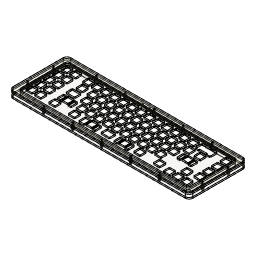
FrogdorCase (Autodesk Fusion 360 design; units mm, degrees)
Autodesk Fusion 360 part; units mm, degrees
(part 1 of 3)
sketch "Frogdor Top Plate" plane through (0, 0, 0) normal (0, 0, 1) x (1, 0, 0)
  line L0 (107.3, -7.3375) -> (107.3, -19.3375)
  line L1 (22.575, -39.3875) -> (34.575, -39.3875)
  arc A0 (184.5, -6.3375) -> (183.5, -7.3375) centre (184.5, -7.3375) ccw
  line L2 (279.75, -6.3375) -> (291.75, -6.3375)
  arc A1 (102.25, -7.3375) -> (101.25, -6.3375) centre (101.25, -7.3375) ccw
  arc A2 (221.6, -19.3375) -> (222.6, -20.3375) centre (222.6, -19.3375) ccw
  arc A3 (183.5, -19.3375) -> (184.5, -20.3375) centre (184.5, -19.3375) ccw
  line L3 (178.45, -7.3375) -> (178.45, -19.3375)
  arc A4 (88.25, -19.3375) -> (89.25, -20.3375) centre (89.25, -19.3375) ccw
  line L4 (184.5, -6.3375) -> (196.5, -6.3375)
  arc A5 (120.3, -20.3375) -> (121.3, -19.3375) centre (120.3, -19.3375) ccw
  arc A6 (196.5, -20.3375) -> (197.5, -19.3375) centre (196.5, -19.3375) ccw
  line L5 (108.3, -6.3375) -> (120.3, -6.3375)
  line L6 (127.35, -6.3375) -> (139.35, -6.3375)
  line L7 (165.45, -6.3375) -> (177.45, -6.3375)
  line L8 (241.65, -6.3375) -> (253.65, -6.3375)
  arc A7 (126.35, -19.3375) -> (127.35, -20.3375) centre (127.35, -19.3375) ccw
  line L9 (145.4, -7.3375) -> (145.4, -19.3375)
  line L10 (317.85, -6.3375) -> (329.85, -6.3375)
  arc A8 (121.3, -7.3375) -> (120.3, -6.3375) centre (120.3, -7.3375) ccw
  arc A9 (146.4, -6.3375) -> (145.4, -7.3375) centre (146.4, -7.3375) ccw
  line L11 (146.4, -6.3375) -> (158.4, -6.3375)
  line L12 (68.9125, -26.3875) -> (68.9125, -38.3875)
  line L13 (146.4, -20.3375) -> (158.4, -20.3375)
  arc A10 (140.35, -7.3375) -> (139.35, -6.3375) centre (139.35, -7.3375) ccw
  arc A11 (145.4, -19.3375) -> (146.4, -20.3375) centre (146.4, -19.3375) ccw
  arc A12 (16.525, -26.3875) -> (15.525, -25.3875) centre (15.525, -26.3875) ccw
  arc A13 (101.25, -20.3375) -> (102.25, -19.3375) centre (101.25, -19.3375) ccw
  line L14 (3.525, -25.3875) -> (15.525, -25.3875)
  line L15 (184.5, -20.3375) -> (196.5, -20.3375)
  arc A14 (178.45, -7.3375) -> (177.45, -6.3375) centre (177.45, -7.3375) ccw
  arc A15 (107.3, -19.3375) -> (108.3, -20.3375) centre (108.3, -19.3375) ccw
  line L16 (127.35, -20.3375) -> (139.35, -20.3375)
  line L17 (126.35, -7.3375) -> (126.35, -19.3375)
  arc A16 (165.45, -6.3375) -> (164.45, -7.3375) centre (165.45, -7.3375) ccw
  line L18 (54.9125, -26.3875) -> (54.9125, -38.3875)
  line L19 (55.9125, -39.3875) -> (67.9125, -39.3875)
  line L20 (197.5, -7.3375) -> (197.5, -19.3375)
  arc A17 (15.525, -39.3875) -> (16.525, -38.3875) centre (15.525, -38.3875) ccw
  line L21 (2.525, -26.3875) -> (2.525, -38.3875)
  arc A18 (164.45, -19.3375) -> (165.45, -20.3375) centre (165.45, -19.3375) ccw
  line L22 (55.9125, -25.3875) -> (67.9125, -25.3875)
  arc A19 (259.7, -19.3375) -> (260.7, -20.3375) centre (260.7, -19.3375) ccw
  arc A20 (159.4, -7.3375) -> (158.4, -6.3375) centre (158.4, -7.3375) ccw
  line L23 (254.65, -7.3375) -> (254.65, -19.3375)
  line L24 (216.55, -7.3375) -> (216.55, -19.3375)
  line L25 (3.525, -39.3875) -> (15.525, -39.3875)
  line L26 (22.575, -25.3875) -> (34.575, -25.3875)
  arc A21 (21.575, -38.3875) -> (22.575, -39.3875) centre (22.575, -38.3875) ccw
  line L27 (329.763, -20.3375) -> (329.85, -20.3375)
  line L28 (164.45, -7.3375) -> (164.45, -19.3375)
  line L29 (165.45, -20.3375) -> (177.45, -20.3375)
  arc A22 (177.45, -20.3375) -> (178.45, -19.3375) centre (177.45, -19.3375) ccw
  line L30 (159.4, -7.3375) -> (159.4, -19.3375)
  line L31 (202.55, -7.3375) -> (202.55, -19.3375)
  line L32 (183.5, -7.3375) -> (183.5, -19.3375)
  line L33 (273.7, -7.3375) -> (273.7, -19.3375)
  line L34 (240.65, -7.3375) -> (240.65, -19.3375)
  arc A23 (279.75, -6.3375) -> (278.75, -7.3375) centre (279.75, -7.3375) ccw
  line L35 (364.1875, -7.3375) -> (364.1875, -19.3375)
  arc A24 (108.3, -6.3375) -> (107.3, -7.3375) centre (108.3, -7.3375) ccw
  arc A25 (89.25, -6.3375) -> (88.25, -7.3375) centre (89.25, -7.3375) ccw
  line L36 (278.75, -7.3375) -> (278.75, -19.3375)
  line L37 (298.8, -20.3375) -> (298.887, -20.3375)
  arc A26 (260.7, -6.3375) -> (259.7, -7.3375) centre (260.7, -7.3375) ccw
  line L38 (351.1875, -6.3375) -> (363.1875, -6.3375)
  line L39 (260.7, -6.3375) -> (272.7, -6.3375)
  arc A27 (291.75, -20.3375) -> (292.75, -19.3375) centre (291.75, -19.3375) ccw
  line L40 (330.85, -7.3375) -> (330.85, -19.3375)
  arc A28 (363.1875, -20.3375) -> (364.1875, -19.3375) centre (363.1875, -19.3375) ccw
  arc A29 (298.8, -6.3375) -> (297.8, -7.3375) centre (298.8, -7.3375) ccw
  arc A30 (297.8, -19.3375) -> (298.8, -20.3375) centre (298.8, -19.3375) ccw
  arc A31 (351.1875, -6.3375) -> (350.1875, -7.3375) centre (351.1875, -7.3375) ccw
  arc A32 (3.525, -25.3875) -> (2.525, -26.3875) centre (3.525, -26.3875) ccw
  arc A33 (254.65, -7.3375) -> (253.65, -6.3375) centre (253.65, -7.3375) ccw
  line L41 (292.75, -7.3375) -> (292.75, -19.3375)
  arc A34 (292.75, -7.3375) -> (291.75, -6.3375) centre (291.75, -7.3375) ccw
  arc A35 (240.65, -19.3375) -> (241.65, -20.3375) centre (241.65, -19.3375) ccw
  arc A36 (278.75, -19.3375) -> (279.75, -20.3375) centre (279.75, -19.3375) ccw
  arc A37 (241.65, -6.3375) -> (240.65, -7.3375) centre (241.65, -7.3375) ccw
  line L42 (351.1875, -20.3375) -> (363.1875, -20.3375)
  line L43 (350.1875, -7.3375) -> (350.1875, -19.3375)
  arc A38 (54.9125, -38.3875) -> (55.9125, -39.3875) centre (55.9125, -38.3875) ccw
  arc A39 (22.575, -25.3875) -> (21.575, -26.3875) centre (22.575, -26.3875) ccw
  arc A40 (168.925, -26.3875) -> (167.925, -25.3875) centre (167.925, -26.3875) ccw
  arc A41 (329.85, -20.3375) -> (330.85, -19.3375) centre (329.85, -19.3375) ccw
  arc A42 (273.7, -7.3375) -> (272.7, -6.3375) centre (272.7, -7.3375) ccw
  arc A43 (253.65, -20.3375) -> (254.65, -19.3375) centre (253.65, -19.3375) ccw
  line L44 (117.825, -39.3875) -> (129.825, -39.3875)
  line L45 (187.975, -26.3875) -> (187.975, -38.3875)
  arc A44 (186.975, -39.3875) -> (187.975, -38.3875) centre (186.975, -38.3875) ccw
  arc A45 (34.575, -39.3875) -> (35.575, -38.3875) centre (34.575, -38.3875) ccw
  line L46 (21.575, -26.3875) -> (21.575, -38.3875)
  line L47 (155.925, -39.3875) -> (167.925, -39.3875)
  line L48 (194.025, -25.3875) -> (206.025, -25.3875)
  line L49 (260.7, -20.3375) -> (272.7, -20.3375)
  arc A46 (194.025, -25.3875) -> (193.025, -26.3875) centre (194.025, -26.3875) ccw
  line L50 (173.975, -26.3875) -> (173.975, -38.3875)
  arc A47 (167.925, -39.3875) -> (168.925, -38.3875) centre (167.925, -38.3875) ccw
  line L51 (207.025, -26.3875) -> (207.025, -38.3875)
  line L52 (130.825, -26.3875) -> (130.825, -38.3875)
  line L53 (259.7, -7.3375) -> (259.7, -19.3375)
  line L54 (98.775, -39.3875) -> (110.775, -39.3875)
  arc A48 (2.525, -38.3875) -> (3.525, -39.3875) centre (3.525, -38.3875) ccw
  line L55 (279.75, -20.3375) -> (291.75, -20.3375)
  arc A49 (155.925, -25.3875) -> (154.925, -26.3875) centre (155.925, -26.3875) ccw
  line L56 (174.975, -25.3875) -> (186.975, -25.3875)
  line L57 (35.575, -26.3875) -> (35.575, -38.3875)
  line L58 (149.875, -26.3875) -> (149.875, -38.3875)
  arc A50 (207.025, -26.3875) -> (206.025, -25.3875) centre (206.025, -26.3875) ccw
  arc A51 (154.925, -38.3875) -> (155.925, -39.3875) centre (155.925, -38.3875) ccw
  line L59 (297.8, -7.3375) -> (297.8, -19.3375)
  arc A52 (330.85, -7.3375) -> (329.85, -6.3375) centre (329.85, -7.3375) ccw
  line L60 (97.775, -26.3875) -> (97.775, -38.3875)
  arc A53 (272.7, -20.3375) -> (273.7, -19.3375) centre (272.7, -19.3375) ccw
  line L61 (16.525, -26.3875) -> (16.525, -38.3875)
  arc A54 (35.575, -26.3875) -> (34.575, -25.3875) centre (34.575, -26.3875) ccw
  arc A55 (350.1875, -19.3375) -> (351.1875, -20.3375) centre (351.1875, -19.3375) ccw
  arc A56 (364.1875, -7.3375) -> (363.1875, -6.3375) centre (363.1875, -7.3375) ccw
  line L62 (98.775, -25.3875) -> (110.775, -25.3875)
  arc A57 (187.975, -26.3875) -> (186.975, -25.3875) centre (186.975, -26.3875) ccw
  line L63 (194.025, -39.3875) -> (206.025, -39.3875)
  arc A58 (129.825, -39.3875) -> (130.825, -38.3875) centre (129.825, -38.3875) ccw
  arc A59 (98.775, -25.3875) -> (97.775, -26.3875) centre (98.775, -26.3875) ccw
  arc A60 (148.875, -39.3875) -> (149.875, -38.3875) centre (148.875, -38.3875) ccw
  line L64 (213.075, -39.3875) -> (225.075, -39.3875)
  line L65 (212.075, -26.3875) -> (212.075, -38.3875)
  line L66 (136.875, -39.3875) -> (148.875, -39.3875)
  line L67 (193.025, -26.3875) -> (193.025, -38.3875)
  line L68 (226.075, -26.3875) -> (226.075, -38.3875)
  line L69 (111.775, -26.3875) -> (111.775, -38.3875)
  line L70 (174.975, -39.3875) -> (186.975, -39.3875)
  arc A61 (55.9125, -25.3875) -> (54.9125, -26.3875) centre (55.9125, -26.3875) ccw
  arc A62 (193.025, -38.3875) -> (194.025, -39.3875) centre (194.025, -38.3875) ccw
  arc A63 (67.9125, -39.3875) -> (68.9125, -38.3875) centre (67.9125, -38.3875) ccw
  arc A64 (117.825, -25.3875) -> (116.825, -26.3875) centre (117.825, -26.3875) ccw
  arc A65 (206.025, -39.3875) -> (207.025, -38.3875) centre (206.025, -38.3875) ccw
  line L71 (79.725, -39.3875) -> (91.725, -39.3875)
  arc A66 (136.875, -25.3875) -> (135.875, -26.3875) centre (136.875, -26.3875) ccw
  line L72 (79.725, -25.3875) -> (91.725, -25.3875)
  line L73 (136.875, -25.3875) -> (148.875, -25.3875)
  arc A67 (78.725, -38.3875) -> (79.725, -39.3875) centre (79.725, -38.3875) ccw
  arc A68 (79.725, -25.3875) -> (78.725, -26.3875) centre (79.725, -26.3875) ccw
  line L74 (116.825, -26.3875) -> (116.825, -38.3875)
  line L75 (154.925, -26.3875) -> (154.925, -38.3875)
  arc A69 (173.975, -38.3875) -> (174.975, -39.3875) centre (174.975, -38.3875) ccw
  line L76 (135.875, -26.3875) -> (135.875, -38.3875)
  arc A70 (110.775, -39.3875) -> (111.775, -38.3875) centre (110.775, -38.3875) ccw
  arc A71 (68.9125, -26.3875) -> (67.9125, -25.3875) centre (67.9125, -26.3875) ccw
  arc A72 (92.725, -26.3875) -> (91.725, -25.3875) centre (91.725, -26.3875) ccw
  arc A73 (130.825, -26.3875) -> (129.825, -25.3875) centre (129.825, -26.3875) ccw
  line L77 (155.925, -25.3875) -> (167.925, -25.3875)
  line L78 (213.075, -25.3875) -> (225.075, -25.3875)
  arc A74 (97.775, -38.3875) -> (98.775, -39.3875) centre (98.775, -38.3875) ccw
  line L79 (117.825, -25.3875) -> (129.825, -25.3875)
  arc A75 (149.875, -26.3875) -> (148.875, -25.3875) centre (148.875, -26.3875) ccw
  arc A76 (111.775, -26.3875) -> (110.775, -25.3875) centre (110.775, -26.3875) ccw
  arc A77 (116.825, -38.3875) -> (117.825, -39.3875) centre (117.825, -38.3875) ccw
  line L80 (92.725, -26.3875) -> (92.725, -38.3875)
  line L81 (168.925, -26.3875) -> (168.925, -38.3875)
  arc A78 (174.975, -25.3875) -> (173.975, -26.3875) centre (174.975, -26.3875) ccw
  arc A79 (263.175, -39.3875) -> (264.175, -38.3875) centre (263.175, -38.3875) ccw
  line L82 (22.575, -58.4375) -> (34.575, -58.4375)
  line L83 (231.125, -26.3875) -> (231.125, -38.3875)
  arc A80 (232.125, -25.3875) -> (231.125, -26.3875) centre (232.125, -26.3875) ccw
  line L84 (232.125, -25.3875) -> (244.125, -25.3875)
  arc A81 (302.275, -26.3875) -> (301.275, -25.3875) centre (301.275, -26.3875) ccw
  arc A82 (269.225, -38.3875) -> (270.225, -39.3875) centre (270.225, -38.3875) ccw
  arc A83 (264.175, -26.3875) -> (263.175, -25.3875) centre (263.175, -26.3875) ccw
  line L85 (264.175, -26.3875) -> (264.175, -38.3875)
  arc A84 (2.525, -57.4375) -> (3.525, -58.4375) centre (3.525, -57.4375) ccw
  arc A85 (288.275, -38.3875) -> (289.275, -39.3875) centre (289.275, -38.3875) ccw
  line L86 (302.275, -26.3875) -> (302.275, -38.3875)
  line L87 (3.525, -58.4375) -> (15.525, -58.4375)
  arc A86 (244.125, -39.3875) -> (245.125, -38.3875) centre (244.125, -38.3875) ccw
  arc A87 (225.075, -39.3875) -> (226.075, -38.3875) centre (225.075, -38.3875) ccw
  arc A88 (212.075, -38.3875) -> (213.075, -39.3875) centre (213.075, -38.3875) ccw
  line L88 (326.0875, -26.3875) -> (326.0875, -38.3875)
  arc A89 (363.1875, -39.3875) -> (364.1875, -38.3875) centre (363.1875, -38.3875) ccw
  line L89 (312.0875, -26.3875) -> (312.0875, -38.3875)
  line L90 (288.275, -26.3875) -> (288.275, -38.3875)
  arc A90 (91.725, -39.3875) -> (92.725, -38.3875) centre (91.725, -38.3875) ccw
  arc A91 (250.175, -38.3875) -> (251.175, -39.3875) centre (251.175, -38.3875) ccw
  line L91 (289.275, -39.3875) -> (301.275, -39.3875)
  arc A92 (245.125, -26.3875) -> (244.125, -25.3875) centre (244.125, -26.3875) ccw
  line L92 (251.175, -25.3875) -> (263.175, -25.3875)
  arc A93 (350.1875, -38.3875) -> (351.1875, -39.3875) centre (351.1875, -38.3875) ccw
  line L93 (2.525, -45.4375) -> (2.525, -57.4375)
  line L94 (232.125, -39.3875) -> (244.125, -39.3875)
  line L95 (35.575, -45.4375) -> (35.575, -57.4375)
  line L96 (251.175, -39.3875) -> (263.175, -39.3875)
  line L97 (3.525, -44.4375) -> (15.525, -44.4375)
  line L98 (313.0875, -25.3875) -> (325.0875, -25.3875)
  line L99 (283.225, -26.3875) -> (283.225, -38.3875)
  arc A94 (351.1875, -25.3875) -> (350.1875, -26.3875) centre (351.1875, -26.3875) ccw
  arc A95 (251.175, -25.3875) -> (250.175, -26.3875) centre (251.175, -26.3875) ccw
  line L100 (270.225, -25.3875) -> (282.225, -25.3875)
  arc A96 (282.225, -39.3875) -> (283.225, -38.3875) centre (282.225, -38.3875) ccw
  arc A97 (289.275, -25.3875) -> (288.275, -26.3875) centre (289.275, -26.3875) ccw
  arc A98 (16.525, -45.4375) -> (15.525, -44.4375) centre (15.525, -45.4375) ccw
  arc A99 (226.075, -26.3875) -> (225.075, -25.3875) centre (225.075, -26.3875) ccw
  line L101 (350.1875, -26.3875) -> (350.1875, -38.3875)
  line L102 (289.275, -25.3875) -> (301.275, -25.3875)
  line L103 (245.125, -26.3875) -> (245.125, -38.3875)
  line L104 (270.225, -39.3875) -> (282.225, -39.3875)
  arc A100 (231.125, -38.3875) -> (232.125, -39.3875) centre (232.125, -38.3875) ccw
  arc A101 (270.225, -25.3875) -> (269.225, -26.3875) centre (270.225, -26.3875) ccw
  line L105 (313.0875, -39.3875) -> (325.0875, -39.3875)
  arc A102 (283.225, -26.3875) -> (282.225, -25.3875) centre (282.225, -26.3875) ccw
  arc A103 (135.875, -38.3875) -> (136.875, -39.3875) centre (136.875, -38.3875) ccw
  line L106 (78.725, -26.3875) -> (78.725, -38.3875)
  arc A104 (326.0875, -26.3875) -> (325.0875, -25.3875) centre (325.0875, -26.3875) ccw
  line L107 (351.1875, -39.3875) -> (363.1875, -39.3875)
  line L108 (22.575, -44.4375) -> (34.575, -44.4375)
  line L109 (250.175, -26.3875) -> (250.175, -38.3875)
  arc A105 (313.0875, -25.3875) -> (312.0875, -26.3875) centre (313.0875, -26.3875) ccw
  line L110 (103.5375, -58.4375) -> (115.5375, -58.4375)
  arc A106 (135.5875, -45.4375) -> (134.5875, -44.4375) centre (134.5875, -45.4375) ccw
  line L111 (141.6375, -44.4375) -> (153.6375, -44.4375)
  arc A107 (364.1875, -26.3875) -> (363.1875, -25.3875) centre (363.1875, -26.3875) ccw
  line L112 (102.5375, -45.4375) -> (102.5375, -57.4375)
  arc A108 (21.575, -57.4375) -> (22.575, -58.4375) centre (22.575, -57.4375) ccw
  arc A109 (115.5375, -58.4375) -> (116.5375, -57.4375) centre (115.5375, -57.4375) ccw
  line L113 (198.7875, -44.4375) -> (210.7875, -44.4375)
  arc A110 (213.075, -25.3875) -> (212.075, -26.3875) centre (213.075, -26.3875) ccw
  line L114 (121.5875, -45.4375) -> (121.5875, -57.4375)
  line L115 (211.7875, -45.4375) -> (211.7875, -57.4375)
  line L116 (52.5313, -45.4375) -> (52.5313, -57.4375)
  line L117 (141.6375, -58.4375) -> (153.6375, -58.4375)
  line L118 (179.7375, -44.4375) -> (191.7375, -44.4375)
  arc A111 (3.525, -44.4375) -> (2.525, -45.4375) centre (3.525, -45.4375) ccw
  line L119 (197.7875, -45.4375) -> (197.7875, -57.4375)
  arc A112 (122.5875, -44.4375) -> (121.5875, -45.4375) centre (122.5875, -45.4375) ccw
  arc A113 (312.0875, -38.3875) -> (313.0875, -39.3875) centre (313.0875, -38.3875) ccw
  line L120 (178.7375, -45.4375) -> (178.7375, -57.4375)
  arc A114 (301.275, -39.3875) -> (302.275, -38.3875) centre (301.275, -38.3875) ccw
  arc A115 (172.6875, -58.4375) -> (173.6875, -57.4375) centre (172.6875, -57.4375) ccw
  line L121 (179.7375, -58.4375) -> (191.7375, -58.4375)
  line L122 (160.6875, -44.4375) -> (172.6875, -44.4375)
  line L123 (103.5375, -44.4375) -> (115.5375, -44.4375)
  arc A116 (52.5312, -57.4375) -> (53.5312, -58.4375) centre (53.5312, -57.4375) ccw
  arc A117 (84.4875, -44.4375) -> (83.4875, -45.4375) centre (84.4875, -45.4375) ccw
  line L124 (84.4875, -58.4375) -> (96.4875, -58.4375)
  line L125 (351.1875, -25.3875) -> (363.1875, -25.3875)
  arc A118 (160.6875, -44.4375) -> (159.6875, -45.4375) centre (160.6875, -45.4375) ccw
  arc A119 (22.575, -44.4375) -> (21.575, -45.4375) centre (22.575, -45.4375) ccw
  arc A120 (154.6375, -45.4375) -> (153.6375, -44.4375) centre (153.6375, -45.4375) ccw
  line L126 (140.6375, -45.4375) -> (140.6375, -57.4375)
  arc A121 (53.5312, -44.4375) -> (52.5312, -45.4375) centre (53.5312, -45.4375) ccw
  arc A122 (116.5375, -45.4375) -> (115.5375, -44.4375) centre (115.5375, -45.4375) ccw
  line L127 (364.1875, -26.3875) -> (364.1875, -38.3875)
  line L128 (135.5875, -45.4375) -> (135.5875, -57.4375)
  arc A123 (15.525, -58.4375) -> (16.525, -57.4375) centre (15.525, -57.4375) ccw
  arc A124 (173.6875, -45.4375) -> (172.6875, -44.4375) centre (172.6875, -45.4375) ccw
  line L129 (122.5875, -58.4375) -> (134.5875, -58.4375)
  line L130 (160.6875, -58.4375) -> (172.6875, -58.4375)
  arc A125 (35.575, -45.4375) -> (34.575, -44.4375) centre (34.575, -45.4375) ccw
  arc A126 (34.575, -58.4375) -> (35.575, -57.4375) centre (34.575, -57.4375) ccw
  line L131 (122.5875, -44.4375) -> (134.5875, -44.4375)
  arc A127 (134.5875, -58.4375) -> (135.5875, -57.4375) centre (134.5875, -57.4375) ccw
  line L132 (173.6875, -45.4375) -> (173.6875, -57.4375)
  arc A128 (121.5875, -57.4375) -> (122.5875, -58.4375) centre (122.5875, -57.4375) ccw
  arc A129 (325.0875, -39.3875) -> (326.0875, -38.3875) centre (325.0875, -38.3875) ccw
  line L133 (16.525, -45.4375) -> (16.525, -57.4375)
  line L134 (83.4875, -45.4375) -> (83.4875, -57.4375)
  arc A130 (102.5375, -57.4375) -> (103.5375, -58.4375) centre (103.5375, -57.4375) ccw
  line L135 (97.4875, -45.4375) -> (97.4875, -57.4375)
  arc A131 (178.7375, -57.4375) -> (179.7375, -58.4375) centre (179.7375, -57.4375) ccw
  line L136 (269.225, -26.3875) -> (269.225, -38.3875)
  arc A132 (179.7375, -44.4375) -> (178.7375, -45.4375) centre (179.7375, -45.4375) ccw
  line L137 (21.575, -45.4375) -> (21.575, -57.4375)
  line L138 (192.7375, -45.4375) -> (192.7375, -57.4375)
  line L139 (198.7875, -58.4375) -> (210.7875, -58.4375)
  arc A133 (97.4875, -45.4375) -> (96.4875, -44.4375) centre (96.4875, -45.4375) ccw
  line L140 (154.6375, -45.4375) -> (154.6375, -57.4375)
  arc A134 (83.4875, -57.4375) -> (84.4875, -58.4375) centre (84.4875, -57.4375) ccw
  line L141 (296.5057, -46.4375) -> (296.5057, -59.4375)
  line L142 (236.8875, -44.4375) -> (248.8875, -44.4375)
  arc A135 (297.5057, -45.4375) -> (296.5057, -46.4375) centre (297.5057, -46.4375) ccw
  line L143 (216.8375, -45.4375) -> (216.8375, -57.4375)
  line L144 (255.9375, -58.4375) -> (267.9375, -58.4375)
  arc A136 (305.9438, -44.4375) -> (304.9438, -45.4375) centre (305.9438, -45.4375) ccw
  arc A137 (302.5057, -60.4375) -> (303.5057, -59.4375) centre (302.5057, -59.4375) ccw
  arc A138 (192.7375, -45.4375) -> (191.7375, -44.4375) centre (191.7375, -45.4375) ccw
  arc A139 (236.8875, -44.4375) -> (235.8875, -45.4375) centre (236.8875, -45.4375) ccw
  line L145 (364.1875, -45.4375) -> (364.1875, -57.4375)
  arc A140 (230.8375, -45.4375) -> (229.8375, -44.4375) centre (229.8375, -45.4375) ccw
  arc A141 (273.9875, -57.4375) -> (274.9875, -58.4375) centre (274.9875, -57.4375) ccw
  arc A142 (317.9438, -58.4375) -> (318.9438, -57.4375) centre (317.9438, -57.4375) ccw
  arc A143 (96.4875, -58.4375) -> (97.4875, -57.4375) centre (96.4875, -57.4375) ccw
  arc A144 (141.6375, -44.4375) -> (140.6375, -45.4375) centre (141.6375, -45.4375) ccw
  arc A145 (140.6375, -57.4375) -> (141.6375, -58.4375) centre (141.6375, -57.4375) ccw
  arc A146 (191.7375, -58.4375) -> (192.7375, -57.4375) centre (191.7375, -57.4375) ccw
  line L146 (303.5057, -46.4375) -> (303.5057, -59.4375)
  arc A147 (286.9875, -58.4375) -> (287.9875, -57.4375) centre (286.9875, -57.4375) ccw
  arc A148 (318.9438, -45.4375) -> (317.9438, -44.4375) centre (317.9438, -45.4375) ccw
  arc A149 (327.3818, -46.4375) -> (326.3818, -45.4375) centre (326.3818, -46.4375) ccw
  line L147 (305.9438, -58.4375) -> (317.9438, -58.4375)
  arc A150 (255.9375, -44.4375) -> (254.9375, -45.4375) centre (255.9375, -45.4375) ccw
  line L148 (236.8875, -58.4375) -> (248.8875, -58.4375)
  arc A151 (268.9375, -45.4375) -> (267.9375, -44.4375) centre (267.9375, -45.4375) ccw
  line L149 (217.8375, -44.4375) -> (229.8375, -44.4375)
  line L150 (297.5057, -60.4375) -> (302.5057, -60.4375)
  line L151 (304.9438, -45.4375) -> (304.9438, -57.4375)
  arc A152 (287.9875, -45.4375) -> (286.9875, -44.4375) centre (286.9875, -45.4375) ccw
  line L152 (235.8875, -45.4375) -> (235.8875, -57.4375)
  arc A153 (103.5375, -44.4375) -> (102.5375, -45.4375) centre (103.5375, -45.4375) ccw
  arc A154 (326.3818, -60.4375) -> (327.3818, -59.4375) centre (326.3818, -59.4375) ccw
  line L153 (217.8375, -58.4375) -> (229.8375, -58.4375)
  arc A155 (159.6875, -57.4375) -> (160.6875, -58.4375) centre (160.6875, -57.4375) ccw
  line L154 (351.1875, -58.4375) -> (363.1875, -58.4375)
  line L155 (327.3818, -46.4375) -> (327.3818, -59.4375)
  arc A156 (217.8375, -44.4375) -> (216.8375, -45.4375) centre (217.8375, -45.4375) ccw
  line L156 (84.4875, -44.4375) -> (96.4875, -44.4375)
  line L157 (318.9438, -45.4375) -> (318.9438, -57.4375)
  arc A157 (320.3818, -59.4375) -> (321.3818, -60.4375) centre (321.3818, -59.4375) ccw
  arc A158 (216.8375, -57.4375) -> (217.8375, -58.4375) centre (217.8375, -57.4375) ccw
  line L158 (297.5057, -45.4375) -> (302.5057, -45.4375)
  arc A159 (197.7875, -57.4375) -> (198.7875, -58.4375) centre (198.7875, -57.4375) ccw
  arc A160 (303.5057, -46.4375) -> (302.5057, -45.4375) centre (302.5057, -46.4375) ccw
  arc A161 (235.8875, -57.4375) -> (236.8875, -58.4375) centre (236.8875, -57.4375) ccw
  arc A162 (296.5057, -59.4375) -> (297.5057, -60.4375) centre (297.5057, -59.4375) ccw
  line L159 (254.9375, -45.4375) -> (254.9375, -57.4375)
  line L160 (305.9438, -44.4375) -> (317.9438, -44.4375)
  line L161 (268.9375, -45.4375) -> (268.9375, -57.4375)
  line L162 (116.5375, -45.4375) -> (116.5375, -57.4375)
  arc A163 (321.3818, -45.4375) -> (320.3818, -46.4375) centre (321.3818, -46.4375) ccw
  arc A164 (153.6375, -58.4375) -> (154.6375, -57.4375) centre (153.6375, -57.4375) ccw
  line L163 (351.1875, -44.4375) -> (363.1875, -44.4375)
  line L164 (159.6875, -45.4375) -> (159.6875, -57.4375)
  line L165 (350.1875, -45.4375) -> (350.1875, -57.4375)
  line L166 (274.9875, -44.4375) -> (286.9875, -44.4375)
  line L167 (287.9875, -45.4375) -> (287.9875, -57.4375)
  line L168 (255.9375, -44.4375) -> (267.9375, -44.4375)
  arc A165 (274.9875, -44.4375) -> (273.9875, -45.4375) centre (274.9875, -45.4375) ccw
  line L169 (249.8875, -45.4375) -> (249.8875, -57.4375)
  arc A166 (249.8875, -45.4375) -> (248.8875, -44.4375) centre (248.8875, -45.4375) ccw
  arc A167 (267.9375, -58.4375) -> (268.9375, -57.4375) centre (267.9375, -57.4375) ccw
  line L170 (321.3818, -45.4375) -> (326.3818, -45.4375)
  arc A168 (54.6183, -64.4875) -> (53.6183, -65.4875) centre (54.6183, -65.4875) ccw
  arc A169 (107.0125, -64.4875) -> (106.0125, -63.4875) centre (106.0125, -64.4875) ccw
  line L171 (84.4942, -65.4875) -> (84.4942, -78.4875)
  line L172 (132.1125, -77.4875) -> (144.1125, -77.4875)
  line L173 (21.575, -64.4875) -> (21.575, -76.4875)
  line L174 (54.6183, -64.4875) -> (59.6183, -64.4875)
  arc A170 (254.9375, -57.4375) -> (255.9375, -58.4375) centre (255.9375, -57.4375) ccw
  line L175 (62.0563, -64.4875) -> (62.0563, -76.4875)
  line L176 (113.0625, -77.4875) -> (125.0625, -77.4875)
  line L177 (107.0125, -64.4875) -> (107.0125, -76.4875)
  line L178 (16.525, -64.4875) -> (16.525, -76.4875)
  arc A171 (76.0563, -64.4875) -> (75.0563, -63.4875) centre (75.0563, -64.4875) ccw
  line L179 (94.0125, -77.4875) -> (106.0125, -77.4875)
  line L180 (22.575, -63.4875) -> (34.575, -63.4875)
  line L181 (273.9875, -45.4375) -> (273.9875, -57.4375)
  arc A172 (112.0625, -76.4875) -> (113.0625, -77.4875) centre (113.0625, -76.4875) ccw
  arc A173 (21.575, -76.4875) -> (22.575, -77.4875) centre (22.575, -76.4875) ccw
  arc A174 (62.0563, -76.4875) -> (63.0562, -77.4875) centre (63.0562, -76.4875) ccw
  line L182 (35.575, -64.4875) -> (35.575, -76.4875)
  line L183 (274.9875, -58.4375) -> (286.9875, -58.4375)
  line L184 (230.8375, -45.4375) -> (230.8375, -57.4375)
  line L185 (320.3818, -46.4375) -> (320.3818, -59.4375)
  arc A175 (125.0625, -77.4875) -> (126.0625, -76.4875) centre (125.0625, -76.4875) ccw
  arc A176 (3.525, -63.4875) -> (2.525, -64.4875) centre (3.525, -64.4875) ccw
  arc A177 (304.9438, -57.4375) -> (305.9438, -58.4375) centre (305.9438, -57.4375) ccw
  arc A178 (229.8375, -58.4375) -> (230.8375, -57.4375) centre (229.8375, -57.4375) ccw
  arc A179 (77.4942, -78.4875) -> (78.4942, -79.4875) centre (78.4942, -78.4875) ccw
  arc A180 (351.1875, -44.4375) -> (350.1875, -45.4375) centre (351.1875, -45.4375) ccw
  line L186 (78.4942, -64.4875) -> (83.4942, -64.4875)
  line L187 (132.1125, -63.4875) -> (144.1125, -63.4875)
  line L188 (63.0562, -63.4875) -> (75.0563, -63.4875)
  arc A181 (248.8875, -58.4375) -> (249.8875, -57.4375) centre (248.8875, -57.4375) ccw
  arc A182 (113.0625, -63.4875) -> (112.0625, -64.4875) centre (113.0625, -64.4875) ccw
  arc A183 (198.7875, -44.4375) -> (197.7875, -45.4375) centre (198.7875, -45.4375) ccw
  arc A184 (126.0625, -64.4875) -> (125.0625, -63.4875) centre (125.0625, -64.4875) ccw
  arc A185 (59.6183, -79.4875) -> (60.6183, -78.4875) centre (59.6183, -78.4875) ccw
  arc A186 (350.1875, -57.4375) -> (351.1875, -58.4375) centre (351.1875, -57.4375) ccw
  line L189 (131.1125, -64.4875) -> (131.1125, -76.4875)
  arc A187 (94.0125, -63.4875) -> (93.0125, -64.4875) centre (94.0125, -64.4875) ccw
  arc A188 (2.525, -76.4875) -> (3.525, -77.4875) centre (3.525, -76.4875) ccw
  line L190 (78.4942, -79.4875) -> (83.4942, -79.4875)
  line L191 (321.3818, -60.4375) -> (326.3818, -60.4375)
  arc A189 (84.4942, -65.4875) -> (83.4942, -64.4875) centre (83.4942, -65.4875) ccw
  arc A190 (15.525, -77.4875) -> (16.525, -76.4875) centre (15.525, -76.4875) ccw
  line L192 (94.0125, -63.4875) -> (106.0125, -63.4875)
  arc A191 (53.6183, -78.4875) -> (54.6183, -79.4875) centre (54.6183, -78.4875) ccw
  arc A192 (22.575, -63.4875) -> (21.575, -64.4875) centre (22.575, -64.4875) ccw
  line L193 (22.575, -77.4875) -> (34.575, -77.4875)
  line L194 (63.0562, -77.4875) -> (75.0563, -77.4875)
  line L195 (76.0563, -64.4875) -> (76.0563, -76.4875)
  line L196 (112.0625, -64.4875) -> (112.0625, -76.4875)
  line L197 (93.0125, -64.4875) -> (93.0125, -76.4875)
  arc A193 (210.7875, -58.4375) -> (211.7875, -57.4375) centre (210.7875, -57.4375) ccw
  line L198 (126.0625, -64.4875) -> (126.0625, -76.4875)
  arc A194 (211.7875, -45.4375) -> (210.7875, -44.4375) centre (210.7875, -45.4375) ccw
  line L199 (2.525, -64.4875) -> (2.525, -76.4875)
  arc A195 (75.0563, -77.4875) -> (76.0563, -76.4875) centre (75.0563, -76.4875) ccw
  line L200 (145.1125, -64.4875) -> (145.1125, -76.4875)
  line L201 (3.525, -63.4875) -> (15.525, -63.4875)
  arc A196 (363.1875, -58.4375) -> (364.1875, -57.4375) centre (363.1875, -57.4375) ccw
  arc A197 (34.575, -77.4875) -> (35.575, -76.4875) centre (34.575, -76.4875) ccw
  arc A198 (93.0125, -76.4875) -> (94.0125, -77.4875) centre (94.0125, -76.4875) ccw
  arc A199 (60.6183, -65.4875) -> (59.6183, -64.4875) centre (59.6183, -65.4875) ccw
  line L202 (60.6183, -65.4875) -> (60.6183, -78.4875)
  arc A200 (201.2625, -77.4875) -> (202.2625, -76.4875) centre (201.2625, -76.4875) ccw
  line L203 (208.3125, -63.4875) -> (220.3125, -63.4875)
  line L204 (53.6183, -65.4875) -> (53.6183, -78.4875)
  arc A201 (164.1625, -64.4875) -> (163.1625, -63.4875) centre (163.1625, -64.4875) ccw
  line L205 (207.3125, -64.4875) -> (207.3125, -76.4875)
  arc A202 (189.2625, -63.4875) -> (188.2625, -64.4875) centre (189.2625, -64.4875) ccw
  arc A203 (208.3125, -63.4875) -> (207.3125, -64.4875) centre (208.3125, -64.4875) ccw
  arc A204 (35.575, -64.4875) -> (34.575, -63.4875) centre (34.575, -64.4875) ccw
  line L206 (208.3125, -77.4875) -> (220.3125, -77.4875)
  line L207 (350.1875, -64.4875) -> (350.1875, -76.4875)
  line L208 (3.525, -77.4875) -> (15.525, -77.4875)
  arc A205 (78.4942, -64.4875) -> (77.4942, -65.4875) centre (78.4942, -65.4875) ccw
  line L209 (183.2125, -64.4875) -> (183.2125, -76.4875)
  line L210 (164.1625, -64.4875) -> (164.1625, -76.4875)
  arc A206 (83.4942, -79.4875) -> (84.4942, -78.4875) centre (83.4942, -78.4875) ccw
  arc A207 (364.1875, -45.4375) -> (363.1875, -44.4375) centre (363.1875, -45.4375) ccw
  line L211 (77.4943, -65.4875) -> (77.4943, -78.4875)
  line L212 (54.6183, -79.4875) -> (59.6183, -79.4875)
  line L213 (151.1625, -77.4875) -> (163.1625, -77.4875)
  arc A208 (245.4125, -76.4875) -> (246.4125, -77.4875) centre (246.4125, -76.4875) ccw
  line L214 (151.1625, -63.4875) -> (163.1625, -63.4875)
  line L215 (245.4125, -64.4875) -> (245.4125, -76.4875)
  line L216 (227.3625, -63.4875) -> (239.3625, -63.4875)
  line L217 (351.1875, -63.4875) -> (363.1875, -63.4875)
  line L218 (364.1875, -64.4875) -> (364.1875, -76.4875)
  arc A209 (246.4125, -63.4875) -> (245.4125, -64.4875) centre (246.4125, -64.4875) ccw
  line L219 (246.4125, -77.4875) -> (258.4125, -77.4875)
  arc A210 (226.3625, -76.4875) -> (227.3625, -77.4875) centre (227.3625, -76.4875) ccw
  line L220 (221.3125, -64.4875) -> (221.3125, -76.4875)
  line L221 (246.4125, -63.4875) -> (258.4125, -63.4875)
  line L222 (202.2625, -64.4875) -> (202.2625, -76.4875)
  arc A211 (202.2625, -64.4875) -> (201.2625, -63.4875) centre (201.2625, -64.4875) ccw
  arc A212 (144.1125, -77.4875) -> (145.1125, -76.4875) centre (144.1125, -76.4875) ccw
  line L223 (169.2125, -64.4875) -> (169.2125, -76.4875)
  line L224 (188.2625, -64.4875) -> (188.2625, -76.4875)
  arc A213 (169.2125, -76.4875) -> (170.2125, -77.4875) centre (170.2125, -76.4875) ccw
  arc A214 (227.3625, -63.4875) -> (226.3625, -64.4875) centre (227.3625, -64.4875) ccw
  arc A215 (264.4625, -76.4875) -> (265.4625, -77.4875) centre (265.4625, -76.4875) ccw
  arc A216 (106.0125, -77.4875) -> (107.0125, -76.4875) centre (106.0125, -76.4875) ccw
  line L225 (150.1625, -64.4875) -> (150.1625, -76.4875)
  line L226 (170.2125, -77.4875) -> (182.2125, -77.4875)
  arc A217 (150.1625, -76.4875) -> (151.1625, -77.4875) centre (151.1625, -76.4875) ccw
  arc A218 (207.3125, -76.4875) -> (208.3125, -77.4875) centre (208.3125, -76.4875) ccw
  arc A219 (163.1625, -77.4875) -> (164.1625, -76.4875) centre (163.1625, -76.4875) ccw
  line L227 (226.3625, -64.4875) -> (226.3625, -76.4875)
  arc A220 (240.3625, -64.4875) -> (239.3625, -63.4875) centre (239.3625, -64.4875) ccw
  line L228 (189.2625, -77.4875) -> (201.2625, -77.4875)
  arc A221 (16.525, -64.4875) -> (15.525, -63.4875) centre (15.525, -64.4875) ccw
  arc A222 (277.4625, -77.4875) -> (278.4625, -76.4875) centre (277.4625, -76.4875) ccw
  line L229 (264.4625, -64.4875) -> (264.4625, -76.4875)
  line L230 (170.2125, -63.4875) -> (182.2125, -63.4875)
  arc A223 (183.2125, -64.4875) -> (182.2125, -63.4875) centre (182.2125, -64.4875) ccw
  arc A224 (170.2125, -63.4875) -> (169.2125, -64.4875) centre (170.2125, -64.4875) ccw
  line L231 (227.3625, -77.4875) -> (239.3625, -77.4875)
  line L232 (265.4625, -77.4875) -> (277.4625, -77.4875)
  arc A225 (131.1125, -76.4875) -> (132.1125, -77.4875) centre (132.1125, -76.4875) ccw
  arc A226 (151.1625, -63.4875) -> (150.1625, -64.4875) centre (151.1625, -64.4875) ccw
  arc A227 (220.3125, -77.4875) -> (221.3125, -76.4875) centre (220.3125, -76.4875) ccw
  arc A228 (259.4125, -64.4875) -> (258.4125, -63.4875) centre (258.4125, -64.4875) ccw
  line L233 (113.0625, -63.4875) -> (125.0625, -63.4875)
  line L234 (351.1875, -77.4875) -> (363.1875, -77.4875)
  arc A229 (63.0562, -63.4875) -> (62.0563, -64.4875) centre (63.0562, -64.4875) ccw
  arc A230 (182.2125, -77.4875) -> (183.2125, -76.4875) centre (182.2125, -76.4875) ccw
  arc A231 (265.4625, -63.4875) -> (264.4625, -64.4875) centre (265.4625, -64.4875) ccw
  line L235 (155.9317, -84.5375) -> (155.9317, -97.5375)
  line L236 (21.575, -83.5375) -> (21.575, -95.5375)
  line L237 (53.5312, -82.5375) -> (65.5312, -82.5375)
  line L238 (278.4625, -64.4875) -> (278.4625, -76.4875)
  line L239 (52.5313, -83.5375) -> (52.5313, -95.5375)
  line L240 (265.4625, -63.4875) -> (277.4625, -63.4875)
  line L241 (22.575, -96.5375) -> (34.575, -96.5375)
  arc A232 (188.2625, -76.4875) -> (189.2625, -77.4875) centre (189.2625, -76.4875) ccw
  line L242 (327.375, -68.25) -> (339.375, -68.25)
  arc A233 (22.575, -82.5375) -> (21.575, -83.5375) centre (22.575, -83.5375) ccw
  arc A234 (15.525, -96.5375) -> (16.525, -95.5375) centre (15.525, -95.5375) ccw
  line L243 (3.525, -96.5375) -> (15.525, -96.5375)
  arc A235 (134.4938, -82.5375) -> (133.4938, -83.5375) centre (134.4938, -83.5375) ccw
  arc A236 (95.3938, -95.5375) -> (96.3938, -96.5375) centre (96.3938, -95.5375) ccw
  line L244 (95.3937, -83.5375) -> (95.3938, -95.5375)
  line L245 (149.9318, -83.5375) -> (154.9318, -83.5375)
  line L246 (240.3625, -64.4875) -> (240.3625, -76.4875)
  line L247 (3.525, -82.5375) -> (15.525, -82.5375)
  line L248 (147.4938, -83.5375) -> (147.4938, -95.5375)
  line L249 (326.375, -69.25) -> (326.375, -81.25)
  line L250 (53.5312, -96.5375) -> (65.5312, -96.5375)
  line L251 (340.375, -69.25) -> (340.375, -81.25)
  arc A237 (239.3625, -77.4875) -> (240.3625, -76.4875) centre (239.3625, -76.4875) ccw
  arc A238 (258.4125, -77.4875) -> (259.4125, -76.4875) centre (258.4125, -76.4875) ccw
  arc A239 (350.1875, -76.4875) -> (351.1875, -77.4875) centre (351.1875, -76.4875) ccw
  arc A240 (340.375, -69.25) -> (339.375, -68.25) centre (339.375, -69.25) ccw
  line L252 (35.575, -83.5375) -> (35.575, -95.5375)
  arc A241 (52.5312, -95.5375) -> (53.5312, -96.5375) centre (53.5312, -95.5375) ccw
  line L253 (189.2625, -63.4875) -> (201.2625, -63.4875)
  arc A242 (3.525, -82.5375) -> (2.525, -83.5375) centre (3.525, -83.5375) ccw
  arc A243 (109.3938, -83.5375) -> (108.3938, -82.5375) centre (108.3938, -83.5375) ccw
  line L254 (2.525, -83.5375) -> (2.525, -95.5375)
  arc A244 (278.4625, -64.4875) -> (277.4625, -63.4875) centre (277.4625, -64.4875) ccw
  line L255 (66.5312, -83.5375) -> (66.5312, -95.5375)
  arc A245 (108.3938, -96.5375) -> (109.3938, -95.5375) centre (108.3938, -95.5375) ccw
  line L256 (96.3938, -82.5375) -> (108.3938, -82.5375)
  arc A246 (339.375, -82.25) -> (340.375, -81.25) centre (339.375, -81.25) ccw
  arc A247 (148.9318, -97.5375) -> (149.9318, -98.5375) centre (149.9318, -97.5375) ccw
  arc A248 (155.9318, -84.5375) -> (154.9318, -83.5375) centre (154.9318, -84.5375) ccw
  arc A249 (65.5312, -96.5375) -> (66.5312, -95.5375) centre (65.5312, -95.5375) ccw
  arc A250 (21.575, -95.5375) -> (22.575, -96.5375) centre (22.575, -95.5375) ccw
  arc A251 (351.1875, -63.4875) -> (350.1875, -64.4875) centre (351.1875, -64.4875) ccw
  arc A252 (133.4938, -95.5375) -> (134.4938, -96.5375) centre (134.4938, -95.5375) ccw
  arc A253 (221.3125, -64.4875) -> (220.3125, -63.4875) centre (220.3125, -64.4875) ccw
  arc A254 (96.3938, -82.5375) -> (95.3938, -83.5375) centre (96.3938, -83.5375) ccw
  arc A255 (132.1125, -63.4875) -> (131.1125, -64.4875) centre (132.1125, -64.4875) ccw
  arc A256 (146.4938, -96.5375) -> (147.4938, -95.5375) centre (146.4938, -95.5375) ccw
  arc A257 (66.5312, -83.5375) -> (65.5312, -82.5375) centre (65.5312, -83.5375) ccw
  arc A258 (34.575, -96.5375) -> (35.575, -95.5375) centre (34.575, -95.5375) ccw
  arc A259 (145.1125, -64.4875) -> (144.1125, -63.4875) centre (144.1125, -64.4875) ccw
  line L257 (132.0557, -84.5375) -> (132.0557, -97.5375)
  line L258 (109.3937, -83.5375) -> (109.3937, -95.5375)
  line L259 (133.4938, -83.5375) -> (133.4938, -95.5375)
  line L260 (259.4125, -64.4875) -> (259.4125, -76.4875)
  line L261 (134.4938, -82.5375) -> (146.4938, -82.5375)
  arc A260 (308.325, -87.3) -> (307.325, -88.3) centre (308.325, -88.3) ccw
  line L262 (204.9313, -83.5375) -> (204.9313, -95.5375)
  line L263 (148.9317, -84.5375) -> (148.9318, -97.5375)
  line L264 (205.9313, -96.5375) -> (217.9313, -96.5375)
  arc A261 (363.1875, -77.4875) -> (364.1875, -76.4875) centre (363.1875, -76.4875) ccw
  line L265 (252.2688, -83.5375) -> (252.2688, -95.5375)
  line L266 (134.4938, -96.5375) -> (146.4938, -96.5375)
  arc A262 (2.525, -95.5375) -> (3.525, -96.5375) centre (3.525, -95.5375) ccw
  arc A263 (16.525, -83.5375) -> (15.525, -82.5375) centre (15.525, -83.5375) ccw
  line L267 (16.525, -83.5375) -> (16.525, -95.5375)
  arc A264 (327.375, -68.25) -> (326.375, -69.25) centre (327.375, -69.25) ccw
  arc A265 (149.9318, -83.5375) -> (148.9318, -84.5375) centre (149.9318, -84.5375) ccw
  arc A266 (154.9318, -98.5375) -> (155.9318, -97.5375) centre (154.9318, -97.5375) ccw
  arc A267 (364.1875, -64.4875) -> (363.1875, -63.4875) centre (363.1875, -64.4875) ccw
  arc A268 (147.4938, -83.5375) -> (146.4938, -82.5375) centre (146.4938, -83.5375) ccw
  line L268 (203.4932, -84.5375) -> (203.4932, -97.5375)
  arc A269 (35.575, -83.5375) -> (34.575, -82.5375) centre (34.575, -83.5375) ccw
  arc A270 (239.2688, -82.5375) -> (238.2688, -83.5375) centre (239.2688, -83.5375) ccw
  line L269 (22.575, -82.5375) -> (34.575, -82.5375)
  line L270 (197.4932, -83.5375) -> (202.4932, -83.5375)
  line L271 (308.325, -87.3) -> (320.325, -87.3)
  arc A271 (238.2688, -95.5375) -> (239.2688, -96.5375) centre (239.2688, -95.5375) ccw
  arc A272 (321.325, -88.3) -> (320.325, -87.3) centre (320.325, -88.3) ccw
  line L272 (149.9318, -98.5375) -> (154.9318, -98.5375)
  line L273 (96.3938, -96.5375) -> (108.3938, -96.5375)
  line L274 (282.1313, -96.5375) -> (294.1313, -96.5375)
  arc A273 (184.5938, -96.5375) -> (185.5938, -95.5375) centre (184.5938, -95.5375) ccw
  line L275 (327.375, -82.25) -> (339.375, -82.25)
  line L276 (196.4933, -84.5375) -> (196.4933, -97.5375)
  arc A274 (53.5312, -82.5375) -> (52.5312, -83.5375) centre (53.5312, -83.5375) ccw
  line L277 (295.1313, -83.5375) -> (295.1313, -95.5375)
  arc A275 (326.375, -81.25) -> (327.375, -82.25) centre (327.375, -81.25) ccw
  line L278 (308.325, -101.3) -> (320.325, -101.3)
  line L279 (205.9313, -82.5375) -> (217.9313, -82.5375)
  line L280 (307.325, -88.3) -> (307.325, -100.3)
  line L281 (346.425, -101.3) -> (358.425, -101.3)
  arc A276 (339.375, -101.3) -> (340.375, -100.3) centre (339.375, -100.3) ccw
  arc A277 (307.325, -100.3) -> (308.325, -101.3) centre (308.325, -100.3) ccw
  line L282 (239.2688, -96.5375) -> (251.2687, -96.5375)
  arc A278 (202.4932, -98.5375) -> (203.4932, -97.5375) centre (202.4932, -97.5375) ccw
  arc A279 (131.0557, -98.5375) -> (132.0557, -97.5375) centre (131.0557, -97.5375) ccw
  line L283 (340.375, -88.3) -> (340.375, -100.3)
  line L284 (239.2688, -82.5375) -> (251.2687, -82.5375)
  line L285 (218.9313, -83.5375) -> (218.9313, -95.5375)
  arc A280 (204.9313, -95.5375) -> (205.9313, -96.5375) centre (205.9313, -95.5375) ccw
  arc A281 (295.1313, -83.5375) -> (294.1313, -82.5375) centre (294.1313, -83.5375) ccw
  arc A282 (282.1313, -82.5375) -> (281.1313, -83.5375) centre (282.1313, -83.5375) ccw
  arc A283 (327.375, -87.3) -> (326.375, -88.3) centre (327.375, -88.3) ccw
  arc A284 (294.1313, -96.5375) -> (295.1313, -95.5375) centre (294.1313, -95.5375) ccw
  arc A285 (252.2687, -83.5375) -> (251.2687, -82.5375) centre (251.2687, -83.5375) ccw
  line L286 (281.1313, -83.5375) -> (281.1313, -95.5375)
  arc A286 (345.425, -100.3) -> (346.425, -101.3) centre (346.425, -100.3) ccw
  line L287 (238.2688, -83.5375) -> (238.2688, -95.5375)
  arc A287 (217.9313, -96.5375) -> (218.9313, -95.5375) centre (217.9313, -95.5375) ccw
  arc A288 (320.325, -101.3) -> (321.325, -100.3) centre (320.325, -100.3) ccw
  arc A289 (197.4932, -83.5375) -> (196.4932, -84.5375) centre (197.4932, -84.5375) ccw
  arc A290 (251.2687, -96.5375) -> (252.2687, -95.5375) centre (251.2687, -95.5375) ccw
  arc A291 (340.375, -88.3) -> (339.375, -87.3) centre (339.375, -88.3) ccw
  arc A292 (218.9313, -83.5375) -> (217.9313, -82.5375) centre (217.9313, -83.5375) ccw
  line L288 (197.4932, -98.5375) -> (202.4932, -98.5375)
  arc A293 (346.425, -87.3) -> (345.425, -88.3) centre (346.425, -88.3) ccw
  arc A294 (203.4932, -84.5375) -> (202.4932, -83.5375) centre (202.4932, -84.5375) ccw
  line L289 (326.375, -88.3) -> (326.375, -100.3)
  arc A295 (205.9313, -82.5375) -> (204.9313, -83.5375) centre (205.9313, -83.5375) ccw
  line L290 (346.425, -87.3) -> (358.425, -87.3)
  line L291 (327.375, -101.3) -> (339.375, -101.3)
  line L292 (185.5938, -83.5375) -> (185.5938, -95.5375)
  arc A296 (185.5937, -83.5375) -> (184.5938, -82.5375) centre (184.5938, -83.5375) ccw
  line L293 (327.375, -87.3) -> (339.375, -87.3)
  line L294 (321.325, -88.3) -> (321.325, -100.3)
  arc A297 (132.0557, -84.5375) -> (131.0557, -83.5375) centre (131.0557, -84.5375) ccw
  line L295 (282.1313, -82.5375) -> (294.1313, -82.5375)
  arc A298 (196.4933, -97.5375) -> (197.4932, -98.5375) centre (197.4932, -97.5375) ccw
  arc A299 (281.1313, -95.5375) -> (282.1313, -96.5375) centre (282.1313, -95.5375) ccw
  arc A300 (326.375, -100.3) -> (327.375, -101.3) centre (327.375, -100.3) ccw
  arc A301 (358.425, -101.3) -> (359.425, -100.3) centre (358.425, -100.3) ccw
  line L296 (120.3312, -84.55) -> (120.3312, -97.55)
  line L297 (166.8313, -83.55) -> (166.8313, -95.55)
  line L298 (71.2938, -45.45) -> (71.2938, -57.45)
  arc A302 (121.3312, -83.55) -> (120.3312, -84.55) centre (121.3312, -84.55) ccw
  arc A303 (120.3312, -97.55) -> (121.3312, -98.55) centre (121.3312, -97.55) ccw
  arc A304 (71.2938, -45.45) -> (70.2938, -44.45) centre (70.2938, -45.45) ccw
  arc A305 (359.425, -88.3) -> (358.425, -87.3) centre (358.425, -88.3) ccw
  arc A306 (166.8313, -95.55) -> (167.8313, -96.55) centre (167.8313, -95.55) ccw
  line L299 (359.425, -88.3) -> (359.425, -100.3)
  arc A307 (70.2938, -58.45) -> (71.2938, -57.45) centre (70.2938, -57.45) ccw
  arc A308 (167.8313, -82.55) -> (166.8313, -83.55) centre (167.8313, -83.55) ccw
  line L300 (345.425, -88.3) -> (345.425, -100.3)
  line L301 (3.525, -20.3375) -> (15.525, -20.3375)
  arc A309 (69.2, -19.3375) -> (70.2, -20.3375) centre (70.2, -19.3375) ccw
  line L302 (69.2, -7.3375) -> (69.2, -19.3375)
  arc A310 (82.2, -20.3375) -> (83.2, -19.3375) centre (82.2, -19.3375) ccw
  arc A311 (2.525, -19.3375) -> (3.525, -20.3375) centre (3.525, -19.3375) ccw
  arc A312 (328.763, -22.325) -> (329.763, -21.325) centre (328.763, -21.325) ccw
  line L303 (323.763, -22.325) -> (328.763, -22.325)
  line L304 (298.887, -20.3375) -> (298.887, -21.325)
  line L305 (3.525, -6.3375) -> (15.525, -6.3375)
  arc A313 (70.2, -6.3375) -> (69.2, -7.3375) centre (70.2, -7.3375) ccw
  arc A314 (83.2, -7.3375) -> (82.2, -6.3375) centre (82.2, -7.3375) ccw
  arc A315 (15.525, -20.3375) -> (16.525, -19.3375) centre (15.525, -19.3375) ccw
  arc A316 (16.525, -7.3375) -> (15.525, -6.3375) centre (15.525, -7.3375) ccw
  arc A317 (35.575, -7.3375) -> (34.575, -6.3375) centre (34.575, -7.3375) ccw
  line L306 (83.2, -7.3375) -> (83.2, -19.3375)
  arc A318 (51.15, -6.3375) -> (50.15, -7.3375) centre (51.15, -7.3375) ccw
  line L307 (299.887, -22.325) -> (304.887, -22.325)
  line L308 (22.575, -20.3375) -> (34.575, -20.3375)
  line L309 (322.763, -20.325) -> (322.763, -21.325)
  arc A319 (64.15, -7.3375) -> (63.15, -6.3375) centre (63.15, -7.3375) ccw
  arc A320 (50.15, -19.3375) -> (51.15, -20.3375) centre (51.15, -19.3375) ccw
  line L310 (21.575, -7.3375) -> (21.575, -19.3375)
  arc A321 (63.15, -20.3375) -> (64.15, -19.3375) centre (63.15, -19.3375) ccw
  line L311 (50.15, -7.3375) -> (50.15, -19.3375)
  arc A322 (22.575, -6.3375) -> (21.575, -7.3375) centre (22.575, -7.3375) ccw
  line L312 (89.25, -6.3375) -> (101.25, -6.3375)
  line L313 (89.25, -20.3375) -> (101.25, -20.3375)
  line L314 (16.525, -7.3375) -> (16.525, -19.3375)
  line L315 (108.3, -20.3375) -> (120.3, -20.3375)
  arc A323 (216.55, -7.3375) -> (215.55, -6.3375) centre (215.55, -7.3375) ccw
  line L316 (222.6, -20.3375) -> (234.6, -20.3375)
  line L317 (235.6, -7.3375) -> (235.6, -19.3375)
  arc A324 (235.6, -7.3375) -> (234.6, -6.3375) centre (234.6, -7.3375) ccw
  arc A325 (21.575, -19.3375) -> (22.575, -20.3375) centre (22.575, -19.3375) ccw
  arc A326 (139.35, -20.3375) -> (140.35, -19.3375) centre (139.35, -19.3375) ccw
  arc A327 (222.6, -6.3375) -> (221.6, -7.3375) centre (222.6, -7.3375) ccw
  line L318 (102.25, -7.3375) -> (102.25, -19.3375)
  line L319 (2.525, -7.3375) -> (2.525, -19.3375)
  line L320 (329.763, -20.3375) -> (329.763, -21.325)
  line L321 (51.15, -20.3375) -> (63.15, -20.3375)
  arc A328 (197.5, -7.3375) -> (196.5, -6.3375) centre (196.5, -7.3375) ccw
  line L322 (22.575, -6.3375) -> (34.575, -6.3375)
  arc A329 (234.6, -20.3375) -> (235.6, -19.3375) centre (234.6, -19.3375) ccw
  arc A330 (3.525, -6.3375) -> (2.525, -7.3375) centre (3.525, -7.3375) ccw
  arc A331 (322.763, -21.325) -> (323.763, -22.325) centre (323.763, -21.325) ccw
  line L323 (70.2, -6.3375) -> (82.2, -6.3375)
  arc A332 (304.887, -22.325) -> (305.887, -21.325) centre (304.887, -21.325) ccw
  line L324 (70.2, -20.3375) -> (82.2, -20.3375)
  line L325 (305.887, -20.325) -> (305.887, -21.325)
  arc A333 (158.4, -20.3375) -> (159.4, -19.3375) centre (158.4, -19.3375) ccw
  line L326 (203.55, -6.3375) -> (215.55, -6.3375)
  arc A334 (34.575, -20.3375) -> (35.575, -19.3375) centre (34.575, -19.3375) ccw
  line L327 (121.3, -7.3375) -> (121.3, -19.3375)
  arc A335 (203.55, -6.3375) -> (202.55, -7.3375) centre (203.55, -7.3375) ccw
  line L328 (35.575, -7.3375) -> (35.575, -19.3375)
  line L329 (203.55, -20.3375) -> (215.55, -20.3375)
  arc A336 (127.35, -6.3375) -> (126.35, -7.3375) centre (127.35, -7.3375) ccw
  arc A337 (202.55, -19.3375) -> (203.55, -20.3375) centre (203.55, -19.3375) ccw
  arc A338 (215.55, -20.3375) -> (216.55, -19.3375) centre (215.55, -19.3375) ccw
  line L330 (222.6, -6.3375) -> (234.6, -6.3375)
  line L331 (221.6, -7.3375) -> (221.6, -19.3375)
  line L332 (140.35, -7.3375) -> (140.35, -19.3375)
  line L333 (241.65, -20.3375) -> (253.65, -20.3375)
  arc A339 (298.887, -21.325) -> (299.887, -22.325) centre (299.887, -21.325) ccw
  line L334 (51.15, -6.3375) -> (63.15, -6.3375)
  line L335 (88.25, -7.3375) -> (88.25, -19.3375)
  line L336 (64.15, -7.3375) -> (64.15, -19.3375)
  line L337 (70.2938, -44.45) -> (53.5312, -44.4375)
  line L338 (70.2938, -58.45) -> (53.5312, -58.4375)
  line L339 (121.3312, -98.55) -> (131.0557, -98.5375)
  line L340 (131.0557, -83.5375) -> (121.3312, -83.55)
  line L341 (167.8313, -82.55) -> (184.5938, -82.5375)
  line L342 (184.5938, -96.5375) -> (167.8313, -96.55)
  line L343 (227.3713, -84.55) -> (227.3713, -97.55)
  arc A340 (226.3313, -98.59) -> (227.3713, -97.55) centre (226.3313, -97.55) ccw
  line L344 (221.3313, -98.59) -> (226.3313, -98.59)
  arc A341 (220.2913, -97.55) -> (221.3313, -98.59) centre (221.3313, -97.55) ccw
  line L345 (220.2912, -84.55) -> (220.2912, -97.55)
  arc A342 (221.3313, -83.51) -> (220.2913, -84.55) centre (221.3313, -84.55) ccw
  line L346 (221.3313, -83.51) -> (226.3313, -83.51)
  arc A343 (227.3713, -84.55) -> (226.3313, -83.51) centre (226.3313, -84.55) ccw
  line L347 (305.887, -20.325) -> (317.6924, -20.325)
  line L348 (317.85, -6.3375) -> (298.8, -6.3375)
  line L349 (317.6924, -20.325) -> (322.763, -20.325)
  arc A344 (379.4175, 0.8925) -> (371.4175, 8.8925) centre (371.4175, 0.8925) ccw
  line L350 (-4.705, 8.8925) -> (371.4175, 8.8925)
  arc A345 (-4.705, 8.8925) -> (-12.705, 0.8925) centre (-4.705, 0.8925) ccw
  line L351 (-12.705, -108.53) -> (-12.705, 0.8925)
  arc A346 (-12.705, -108.53) -> (-4.705, -116.53) centre (-4.705, -108.53) ccw
  line L352 (371.4175, -116.53) -> (-4.705, -116.53)
  arc A347 (371.4175, -116.53) -> (379.4175, -108.53) centre (371.4175, -108.53) ccw
  line L353 (379.4175, 0.8925) -> (379.4175, -108.53)
  circle A348 centre (56.982, 3.3925) radius 1.55
  circle A349 centre (120.1693, 3.3925) radius 1.55
  circle A350 centre (183.3563, 3.3925) radius 1.55
  circle A351 centre (246.5433, 3.3925) radius 1.55
  circle A352 centre (309.7305, 3.3925) radius 1.55
  circle A353 centre (373.9175, -25.7132) radius 1.55
  circle A354 centre (373.9175, -81.9243) radius 1.55
  circle A355 centre (309.7305, -111.03) radius 1.55
  circle A356 centre (246.5433, -111.03) radius 1.55
  circle A357 centre (183.3563, -111.03) radius 1.55
  circle A358 centre (120.1693, -111.03) radius 1.55
  circle A359 centre (56.982, -111.03) radius 1.55
  circle A360 centre (-7.205, -81.9243) radius 1.55
  circle A361 centre (-7.205, -25.7132) radius 1.55
  point P0 (183.3563, 3.3925)
  point P1 (246.5433, 3.3925)
  point P2 (309.7305, 3.3925)
  point P3 (373.9175, -25.7132)
  point P4 (373.9175, -81.9243)
  point P5 (309.7305, -111.03)
  point P6 (246.5433, -111.03)
  point P7 (183.3563, -111.03)
  point P8 (120.1693, -111.03)
  point P9 (56.982, -111.03)
  point P10 (-7.205, -81.9243)
  point P11 (-7.205, -25.7132)
  point P12 (56.982, 3.3925)
  point P13 (120.1693, 3.3925)
  dimension "d99" = 3.1
  dimension "d100" = 3.1
  dimension "d101" = 3.1
  dimension "d102" = 3.1
  dimension "d103" = 3.1
  dimension "d104" = 3.1
  dimension "d105" = 3.1
  dimension "d106" = 3.1
  dimension "d107" = 3.1
  dimension "d108" = 3.1